Autodesk Inventor part; units mm, degrees
(part 2 of 2)
sketch "スケッチ6" plane through (0, 0, -3) normal (0, 0, -1) x (-1, 0, 0)
  line L0 (6.4129, 87.5325) -> (28.1361, 63.912) projected
  arc A0 (28.2548, 62.7161) -> (28.1361, 63.912) centre (27.4001, 63.2351) ccw projected
  arc A1 (28.2548, 62.7161) -> (28.3025, 54.3338) centre (35.0928, 58.5637) ccw projected
  arc A2 (28.2815, 53.244) -> (28.3025, 54.3338) centre (27.4537, 53.805) ccw projected
  arc A3 (28.2815, 53.244) -> (27.9209, 52.5865) centre (31.5928, 51) ccw projected
  arc A4 (26.9209, 51.9865) -> (27.9209, 52.5865) centre (27.0029, 52.9832) ccw projected
  arc A5 (26.9209, 51.9865) -> (24.1928, 51.2) centre (26.5928, 48) ccw projected
  arc A6 (23.5928, 51) -> (24.1928, 51.2) centre (23.5928, 52) ccw projected
  line L1 (23.5928, 51) -> (-14.9001, 51) projected
  arc A7 (-15.5001, 51.2) -> (-14.9001, 51) centre (-14.9001, 52) ccw projected
  arc A8 (-15.5001, 51.2) -> (-18.2282, 51.9865) centre (-17.9001, 48) ccw projected
  arc A9 (-19.2282, 52.5865) -> (-18.2282, 51.9865) centre (-18.3102, 52.9832) ccw projected
  arc A10 (-19.2282, 52.5865) -> (-20.5352, 54.226) centre (-22.9001, 51) ccw projected
  arc A11 (-20.7229, 55.6596) -> (-20.5352, 54.226) centre (-19.944, 55.0325) ccw projected
  line L2 (-20.7229, 55.6596) -> (4.8979, 87.4826) projected
  arc A12 (6.4129, 87.5325) -> (4.8979, 87.4826) centre (5.6769, 86.8555) ccw projected
  line L3 (3.033, 89.9501) -> (-23.1212, 57.4646) projected
  arc A13 (-24.9001, 58.0917) -> (-23.1212, 57.4646) centre (-23.9001, 58.0917) ccw projected
  line L4 (-24.9001, 58.0917) -> (-24.9001, 116.7814) projected
  arc A14 (-24.1779, 117.742) -> (-24.9001, 116.7814) centre (-23.9001, 116.7814) ccw projected
  arc A15 (-24.1779, 117.742) -> (-22.8335, 118.2662) centre (-26.4001, 125.4272) ccw projected
  arc A16 (-21.6516, 118.048) -> (-22.8335, 118.2662) centre (-22.3876, 117.3711) ccw projected
  line L5 (-21.6516, 118.048) -> (2.9902, 91.2541) projected
  arc A17 (3.033, 89.9501) -> (2.9902, 91.2541) centre (2.2541, 90.5772) ccw projected
  arc A18 (10.5684, 93.4279) -> (14.253, 93.0788) centre (13.05, 100) ccw projected
  arc A19 (15.3071, 92.5632) -> (14.253, 93.0788) centre (14.4242, 92.0935) ccw projected
  line L6 (15.3071, 92.5632) -> (24.5983, 75.0975) projected
  arc A20 (22.9794, 73.9509) -> (24.5983, 75.0975) centre (23.7154, 74.6278) ccw projected
  line L7 (22.9794, 73.9509) -> (8.1117, 90.1171) projected
  arc A21 (8.0688, 91.4211) -> (8.1117, 90.1171) centre (8.8478, 90.794) ccw projected
  line L8 (8.0688, 91.4211) -> (9.4362, 93.1195) projected
  arc A22 (10.5684, 93.4279) -> (9.4362, 93.1195) centre (10.2151, 92.4924) ccw projected
  line L9 (-14.28, 117.3918) -> (-15.0025, 116.7273) projected
  arc A23 (-16.4155, 116.7864) -> (-15.0025, 116.7273) centre (-15.6794, 117.4633) ccw projected
  line L10 (-16.4155, 116.7864) -> (-18.5628, 119.1212) projected
  arc A24 (-17.4982, 120.7426) -> (-18.5628, 119.1212) centre (-17.8267, 119.7981) ccw projected
  line L11 (-17.4982, 120.7426) -> (-14.7786, 119.7967) projected
  arc A25 (-14.1165, 118.9889) -> (-14.7786, 119.7967) centre (-15.1071, 118.8522) ccw projected
  arc A26 (-14.1165, 118.9889) -> (-13.9936, 118.3962) centre (-9.6587, 119.604) ccw projected
  arc A27 (-14.28, 117.3918) -> (-13.9936, 118.3962) centre (-14.9569, 118.1278) ccw projected
  arc A28 (32.5928, 51) -> (30.5928, 51) centre (31.5928, 51) ccw projected
  line L12 (32.5928, 51) -> (37.5928, 51) projected
  arc A29 (39.5928, 51) -> (37.5928, 51) centre (38.5928, 51) ccw projected
  line L13 (39.5928, 51) -> (39.5928, 48) projected
  arc A30 (37.5928, 48) -> (39.5928, 48) centre (38.5928, 48) ccw projected
  line L14 (37.5928, 48) -> (32.5928, 48) projected
  arc A31 (30.5928, 48) -> (32.5928, 48) centre (31.5928, 48) ccw projected
  line L15 (30.5928, 48) -> (30.5928, 51) projected
  circle A32 centre (-9.6587, 119.604) radius 1.5 projected
  circle A33 centre (13.05, 100) radius 4.025 projected
  circle A34 centre (-26.4001, 125.4272) radius 4 projected
  circle A35 centre (35.0928, 58.5637) radius 4 projected
  line L16 (7.0994, 95.0009) -> (6.2039, 93.8886) projected
  arc A36 (4.689, 93.8388) -> (6.2039, 93.8886) centre (5.425, 94.5157) ccw projected
  line L17 (4.689, 93.8388) -> (-13.0309, 113.1062) projected
  arc A37 (-12.9717, 114.5191) -> (-13.0309, 113.1062) centre (-12.2948, 113.7831) ccw projected
  line L18 (-12.9717, 114.5191) -> (-12.2492, 115.1836) projected
  arc A38 (-11.2244, 115.3851) -> (-12.2492, 115.1836) centre (-11.5723, 114.4476) ccw projected
  arc A39 (-11.2244, 115.3851) -> (-7.9613, 115.4364) centre (-9.6587, 119.604) ccw projected
  arc A40 (-6.9306, 115.2672) -> (-7.9613, 115.4364) centre (-7.5841, 114.5103) ccw projected
  line L19 (-6.9306, 115.2672) -> (6.2975, 103.8477) projected
  arc A41 (6.5669, 102.7056) -> (6.2975, 103.8477) centre (5.644, 103.0907) ccw projected
  arc A42 (6.5669, 102.7056) -> (7.1591, 96.1728) centre (13.05, 100) ccw projected
  arc A43 (7.0994, 95.0009) -> (7.1591, 96.1728) centre (6.3205, 95.628) ccw projected
  arc A44 (-28.9001, 51) -> (-30.9001, 51) centre (-29.9001, 51) ccw projected
  line L20 (-28.9001, 51) -> (-23.9001, 51) projected
  arc A45 (-21.9001, 51) -> (-23.9001, 51) centre (-22.9001, 51) ccw projected
  line L21 (-21.9001, 51) -> (-21.9001, 48) projected
  arc A46 (-23.9001, 48) -> (-21.9001, 48) centre (-22.9001, 48) ccw projected
  line L22 (-23.9001, 48) -> (-28.9001, 48) projected
  arc A47 (-30.9001, 48) -> (-28.9001, 48) centre (-29.9001, 48) ccw projected
  line L23 (-30.9001, 48) -> (-30.9001, 51) projected
  line L24 (-27.9001, 116.7814) -> (-27.9001, 55.899) projected
  arc A48 (-29.1001, 54.9192) -> (-27.9001, 55.899) centre (-28.9001, 55.899) ccw projected
  arc A49 (-29.1001, 54.9192) -> (-33.572, 52.5865) centre (-29.9001, 51) ccw projected
  arc A50 (-34.572, 51.9865) -> (-33.572, 52.5865) centre (-34.49, 52.9832) ccw projected
  arc A51 (-34.572, 51.9865) -> (-37.3001, 51.2) centre (-34.9001, 48) ccw projected
  arc A52 (-37.9001, 51) -> (-37.3001, 51.2) centre (-37.9001, 52) ccw projected
  line L25 (-37.9001, 51) -> (-38.9001, 51) projected
  line L26 (-38.9001, 51) -> (-38.9001, 48) projected
  line L27 (-38.9001, 48) -> (-35.9001, 48) projected
  arc A53 (-33.9001, 48) -> (-35.9001, 48) centre (-34.9001, 48) ccw projected
  line L28 (-33.9001, 48) -> (-33.9001, 45) projected
  line L29 (-33.9001, 45) -> (-18.9001, 45) projected
  line L30 (-18.9001, 45) -> (-18.9001, 48) projected
  arc A54 (-16.9001, 48) -> (-18.9001, 48) centre (-17.9001, 48) ccw projected
  line L31 (-16.9001, 48) -> (25.5928, 48) projected
  arc A55 (27.5928, 48) -> (25.5928, 48) centre (26.5928, 48) ccw projected
  line L32 (27.5928, 48) -> (27.5928, 45) projected
  line L33 (27.5928, 45) -> (42.5928, 45) projected
  line L34 (42.5928, 45) -> (42.5928, 48) projected
  arc A56 (44.5928, 48) -> (42.5928, 48) centre (43.5928, 48) ccw projected
  line L35 (44.5928, 48) -> (47.5928, 48) projected
  line L36 (47.5928, 48) -> (47.5928, 51) projected
  line L37 (47.5928, 51) -> (46.5928, 51) projected
  arc A57 (45.9928, 51.2) -> (46.5928, 51) centre (46.5928, 52) ccw projected
  arc A58 (45.9928, 51.2) -> (43.2647, 51.9865) centre (43.5928, 48) ccw projected
  arc A59 (42.2647, 52.5865) -> (43.2647, 51.9865) centre (43.1827, 52.9832) ccw projected
  arc A60 (42.2647, 52.5865) -> (41.904, 53.244) centre (38.5928, 51) ccw projected
  arc A61 (41.883, 54.3338) -> (41.904, 53.244) centre (42.7318, 53.805) ccw projected
  arc A62 (41.883, 54.3338) -> (33.4453, 66.3922) centre (35.0928, 58.5637) ccw projected
  arc A63 (32.3566, 66.9011) -> (33.4453, 66.3922) centre (33.2394, 67.3708) ccw projected
  line L38 (32.3566, 66.9011) -> (17.9557, 93.9721) projected
  arc A64 (18.1172, 95.1344) -> (17.9557, 93.9721) centre (18.8385, 94.4418) ccw projected
  arc A65 (18.1172, 95.1344) -> (9.4271, 106.0187) centre (13.05, 100) ccw projected
  arc A66 (8.2579, 106.1185) -> (9.4271, 106.0187) centre (8.9114, 106.8755) ccw projected
  line L39 (8.2579, 106.1185) -> (-4.9702, 117.5381) projected
  arc A67 (-5.288, 118.533) -> (-4.9702, 117.5381) centre (-4.3167, 118.295) ccw projected
  arc A68 (-5.288, 118.533) -> (-12.7725, 122.8527) centre (-9.6587, 119.604) ccw projected
  arc A69 (-13.793, 122.6301) -> (-12.7725, 122.8527) centre (-13.4645, 123.5746) ccw projected
  line L40 (-13.793, 122.6301) -> (-17.7414, 124.0035) projected
  arc A70 (-18.4115, 125.0013) -> (-17.7414, 124.0035) centre (-17.4129, 124.948) ccw projected
  arc A71 (-18.4115, 125.0013) -> (-28.6223, 117.742) centre (-26.4001, 125.4272) ccw projected
  arc A72 (-27.9001, 116.7814) -> (-28.6223, 117.742) centre (-28.9001, 116.7814) ccw projected
  circle A73 centre (-9.6587, 119.604) radius 1.5 projected
  circle A74 centre (-9.6587, 119.604) radius 3
  point P0 (0, 0)
  dimension "d89" = 6
  constraints: 1 centre point, 1 coincident
  measures "d89" diameter of A74
extrude "押し出し7" cut sketch "スケッチ6" against normal blind 0.6 contours A74
sketch "スケッチ7" plane through (-35.0928, 58.5637, -2.3) normal (0, 0, -1) x (-1, 0, 0)
  arc A0 (6.7903, -4.2299) -> (6.8112, -5.3197) centre (7.6391, -4.7587) ccw projected
  arc A1 (7.1719, -5.9772) -> (6.8112, -5.3197) centre (3.5, -7.5637) ccw projected
  arc A2 (7.1719, -5.9772) -> (8.1719, -6.5772) centre (8.0899, -5.5805) ccw projected
  arc A3 (10.9, -7.3637) -> (8.1719, -6.5772) centre (8.5, -10.5637) ccw projected
  arc A4 (10.9, -7.3637) -> (11.5, -7.5637) centre (11.5, -6.5637) ccw projected
  line L0 (11.5, -7.5637) -> (12.5, -7.5637) projected
  line L1 (12.5, -7.5637) -> (12.5, -10.5637) projected
  line L2 (12.5, -10.5637) -> (9.5, -10.5637) projected
  arc A5 (9.5, -10.5637) -> (7.5, -10.5637) centre (8.5, -10.5637) ccw projected
  line L3 (7.5, -10.5637) -> (7.5, -13.5637) projected
  line L4 (7.5, -13.5637) -> (-7.5, -13.5637) projected
  line L5 (-7.5, -13.5637) -> (-7.5, -10.5637) projected
  arc A6 (-7.5, -10.5637) -> (-9.5, -10.5637) centre (-8.5, -10.5637) ccw projected
  line L6 (-9.5, -10.5637) -> (-51.9929, -10.5637) projected
  arc A7 (-51.9929, -10.5637) -> (-53.9929, -10.5637) centre (-52.9929, -10.5637) ccw projected
  line L7 (-53.9929, -10.5637) -> (-53.9929, -13.5637) projected
  line L8 (-53.9929, -13.5637) -> (-68.9929, -13.5637) projected
  line L9 (-68.9929, -13.5637) -> (-68.9929, -10.5637) projected
  arc A8 (-68.9929, -10.5637) -> (-70.9929, -10.5637) centre (-69.9929, -10.5637) ccw projected
  line L10 (-70.9929, -10.5637) -> (-73.9929, -10.5637) projected
  line L11 (-73.9929, -10.5637) -> (-73.9929, -7.5637) projected
  line L12 (-73.9929, -7.5637) -> (-72.9929, -7.5637) projected
  arc A9 (-72.9929, -7.5637) -> (-72.3929, -7.3637) centre (-72.9929, -6.5637) ccw projected
  arc A10 (-69.6648, -6.5772) -> (-72.3929, -7.3637) centre (-69.9929, -10.5637) ccw projected
  arc A11 (-69.6648, -6.5772) -> (-68.6648, -5.9772) centre (-69.5828, -5.5805) ccw projected
  arc A12 (-64.1929, -3.6445) -> (-68.6648, -5.9772) centre (-64.9929, -7.5637) ccw projected
  arc A13 (-64.1929, -3.6445) -> (-62.9929, -2.6647) centre (-63.9929, -2.6647) ccw projected
  line L13 (-62.9929, -2.6647) -> (-62.9929, 58.2177) projected
  arc A14 (-62.9929, 58.2177) -> (-63.7151, 59.1783) centre (-63.9929, 58.2177) ccw projected
  arc A15 (-53.5042, 66.4376) -> (-63.7151, 59.1783) centre (-61.4929, 66.8635) ccw projected
  arc A16 (-53.5042, 66.4376) -> (-52.8342, 65.4398) centre (-52.5057, 66.3843) ccw projected
  line L14 (-52.8342, 65.4398) -> (-48.8858, 64.0664) projected
  arc A17 (-48.8858, 64.0664) -> (-47.8653, 64.289) centre (-48.5572, 65.0109) ccw projected
  arc A18 (-40.3808, 59.9693) -> (-47.8653, 64.289) centre (-44.7515, 61.0403) ccw projected
  arc A19 (-40.3808, 59.9693) -> (-40.063, 58.9744) centre (-39.4095, 59.7313) ccw projected
  line L15 (-40.063, 58.9744) -> (-26.8349, 47.5548) projected
  arc A20 (-26.8349, 47.5548) -> (-25.6657, 47.455) centre (-26.1814, 48.3118) ccw projected
  arc A21 (-16.9756, 36.5707) -> (-25.6657, 47.455) centre (-22.0428, 41.4363) ccw projected
  arc A22 (-16.9756, 36.5707) -> (-17.1371, 35.4084) centre (-16.2543, 35.8781) ccw projected
  line L16 (-17.1371, 35.4084) -> (-2.7362, 8.3375) projected
  arc A23 (-2.7362, 8.3375) -> (-1.6474, 7.8285) centre (-1.8534, 8.8071) ccw projected
  arc A24 (6.7903, -4.2299) -> (-1.6474, 7.8285) centre (0, 0) ccw projected
  arc A25 (-24.5244, 34.8642) -> (-25.6566, 34.5558) centre (-24.8776, 33.9287) ccw projected
  line L17 (-25.6566, 34.5558) -> (-27.0239, 32.8574) projected
  arc A26 (-27.0239, 32.8574) -> (-26.9811, 31.5534) centre (-26.245, 32.2303) ccw projected
  line L18 (-26.9811, 31.5534) -> (-12.1134, 15.3872) projected
  arc A27 (-12.1134, 15.3872) -> (-10.4945, 16.5338) centre (-11.3773, 16.0642) ccw projected
  line L19 (-10.4945, 16.5338) -> (-19.7857, 33.9995) projected
  arc A28 (-19.7857, 33.9995) -> (-20.8398, 34.5151) centre (-20.6685, 33.5298) ccw projected
  arc A29 (-24.5244, 34.8642) -> (-20.8398, 34.5151) centre (-22.0428, 41.4363) ccw projected
  arc A30 (-59.2707, 59.1783) -> (-59.9929, 58.2177) centre (-58.9929, 58.2177) ccw projected
  line L20 (-59.9929, 58.2177) -> (-59.9929, -0.472) projected
  arc A31 (-59.9929, -0.472) -> (-58.214, -1.0991) centre (-58.9929, -0.472) ccw projected
  line L21 (-58.214, -1.0991) -> (-32.0597, 31.3864) projected
  arc A32 (-32.0597, 31.3864) -> (-32.1026, 32.6904) centre (-32.8387, 32.0135) ccw projected
  line L22 (-32.1026, 32.6904) -> (-56.7444, 59.4843) projected
  arc A33 (-56.7444, 59.4843) -> (-57.9263, 59.7025) centre (-57.4804, 58.8074) ccw projected
  arc A34 (-59.2707, 59.1783) -> (-57.9263, 59.7025) centre (-61.4929, 66.8635) ccw projected
  arc A35 (-28.6799, 28.9688) -> (-30.1948, 28.9189) centre (-29.4159, 28.2918) ccw projected
  line L23 (-30.1948, 28.9189) -> (-55.8157, -2.9041) projected
  arc A36 (-55.8157, -2.9041) -> (-55.628, -4.3377) centre (-55.0367, -3.5312) ccw projected
  arc A37 (-54.321, -5.9772) -> (-55.628, -4.3377) centre (-57.9929, -7.5637) ccw projected
  arc A38 (-54.321, -5.9772) -> (-53.321, -6.5772) centre (-53.403, -5.5805) ccw projected
  arc A39 (-50.5929, -7.3637) -> (-53.321, -6.5772) centre (-52.9929, -10.5637) ccw projected
  arc A40 (-50.5929, -7.3637) -> (-49.9929, -7.5637) centre (-49.9929, -6.5637) ccw projected
  line L24 (-49.9929, -7.5637) -> (-11.5, -7.5637) projected
  arc A41 (-11.5, -7.5637) -> (-10.9, -7.3637) centre (-11.5, -6.5637) ccw projected
  arc A42 (-8.1719, -6.5772) -> (-10.9, -7.3637) centre (-8.5, -10.5637) ccw projected
  arc A43 (-8.1719, -6.5772) -> (-7.1719, -5.9772) centre (-8.0899, -5.5805) ccw projected
  arc A44 (-6.8112, -5.3197) -> (-7.1719, -5.9772) centre (-3.5, -7.5637) ccw projected
  arc A45 (-6.8112, -5.3197) -> (-6.7903, -4.2299) centre (-7.6391, -4.7587) ccw projected
  arc A46 (-6.838, 4.1524) -> (-6.7903, -4.2299) centre (0, 0) ccw projected
  arc A47 (-6.838, 4.1524) -> (-6.9567, 5.3483) centre (-7.6927, 4.6714) ccw projected
  line L25 (-6.9567, 5.3483) -> (-28.6799, 28.9688) projected
  line L26 (2.5, -7.5637) -> (-2.5, -7.5637) projected
  arc A48 (-2.5, -7.5637) -> (-4.5, -7.5637) centre (-3.5, -7.5637) ccw projected
  line L27 (-4.5, -7.5637) -> (-4.5, -10.5637) projected
  arc A49 (-4.5, -10.5637) -> (-2.5, -10.5637) centre (-3.5, -10.5637) ccw projected
  line L28 (-2.5, -10.5637) -> (2.5, -10.5637) projected
  arc A50 (2.5, -10.5637) -> (4.5, -10.5637) centre (3.5, -10.5637) ccw projected
  line L29 (4.5, -10.5637) -> (4.5, -7.5637) projected
  arc A51 (4.5, -7.5637) -> (2.5, -7.5637) centre (3.5, -7.5637) ccw projected
  line L30 (-58.9929, -7.5637) -> (-63.9929, -7.5637) projected
  arc A52 (-63.9929, -7.5637) -> (-65.9929, -7.5637) centre (-64.9929, -7.5637) ccw projected
  line L31 (-65.9929, -7.5637) -> (-65.9929, -10.5637) projected
  arc A53 (-65.9929, -10.5637) -> (-63.9929, -10.5637) centre (-64.9929, -10.5637) ccw projected
  line L32 (-63.9929, -10.5637) -> (-58.9929, -10.5637) projected
  arc A54 (-58.9929, -10.5637) -> (-56.9929, -10.5637) centre (-57.9929, -10.5637) ccw projected
  line L33 (-56.9929, -10.5637) -> (-56.9929, -7.5637) projected
  arc A55 (-56.9929, -7.5637) -> (-58.9929, -7.5637) centre (-57.9929, -7.5637) ccw projected
  arc A56 (-46.3171, 56.8214) -> (-47.342, 56.6199) centre (-46.665, 55.8839) ccw projected
  line L34 (-47.342, 56.6199) -> (-48.0645, 55.9554) projected
  arc A57 (-48.0645, 55.9554) -> (-48.1236, 54.5425) centre (-47.3876, 55.2194) ccw projected
  line L35 (-48.1236, 54.5425) -> (-30.4038, 35.2751) projected
  arc A58 (-30.4038, 35.2751) -> (-28.8888, 35.3249) centre (-29.6678, 35.952) ccw projected
  line L36 (-28.8888, 35.3249) -> (-27.9933, 36.4372) projected
  arc A59 (-27.9933, 36.4372) -> (-27.9337, 37.6091) centre (-28.7723, 37.0643) ccw projected
  arc A60 (-28.5259, 44.1419) -> (-27.9337, 37.6091) centre (-22.0428, 41.4363) ccw projected
  arc A61 (-28.5259, 44.1419) -> (-28.7953, 45.284) centre (-29.4487, 44.527) ccw projected
  line L37 (-28.7953, 45.284) -> (-42.0234, 56.7035) projected
  arc A62 (-42.0234, 56.7035) -> (-43.054, 56.8727) centre (-42.6768, 55.9466) ccw projected
  arc A63 (-46.3171, 56.8214) -> (-43.054, 56.8727) centre (-44.7515, 61.0403) ccw projected
  arc A64 (-52.591, 62.1789) -> (-53.6555, 60.5575) centre (-52.9195, 61.2344) ccw projected
  line L38 (-53.6555, 60.5575) -> (-51.5083, 58.2227) projected
  arc A65 (-51.5083, 58.2227) -> (-50.0953, 58.1636) centre (-50.7722, 58.8996) ccw projected
  line L39 (-50.0953, 58.1636) -> (-49.3728, 58.8281) projected
  arc A66 (-49.3728, 58.8281) -> (-49.0864, 59.8325) centre (-50.0497, 59.5641) ccw projected
  arc A67 (-49.2092, 60.4252) -> (-49.0864, 59.8325) centre (-44.7515, 61.0403) ccw projected
  arc A68 (-49.2092, 60.4252) -> (-49.8713, 61.233) centre (-50.1999, 60.2885) ccw projected
  line L40 (-49.8713, 61.233) -> (-52.591, 62.1789) projected
  circle A69 centre (0, 0) radius 4 projected
  circle A70 centre (-61.4929, 66.8635) radius 4 projected
  circle A71 centre (-61.4929, 66.8635) radius 2 projected
  circle A72 centre (0, 0) radius 2 projected
  circle A73 centre (-22.0428, 41.4363) radius 4.025 projected
  circle A74 centre (-44.7515, 61.0403) radius 1.5 projected
  point P0 (-35.0928, -58.5637)
extrude "押し出し8" cut sketch "スケッチ7" against normal blind 0.5 contours A69 | A70
sketch "スケッチ8" plane through (0, 0, -3) normal (0, 0, -1) x (-1, 0, 0)
  circle A0 centre (-9.6587, 119.604) radius 3 projected
  arc A1 (41.883, 54.3338) -> (41.904, 53.244) centre (42.7318, 53.805) ccw projected
  arc A2 (42.2647, 52.5865) -> (41.904, 53.244) centre (38.5928, 51) ccw projected
  arc A3 (42.2647, 52.5865) -> (43.2647, 51.9865) centre (43.1827, 52.9832) ccw projected
  arc A4 (45.9928, 51.2) -> (43.2647, 51.9865) centre (43.5928, 48) ccw projected
  arc A5 (45.9928, 51.2) -> (46.5928, 51) centre (46.5928, 52) ccw projected
  line L0 (46.5928, 51) -> (47.5928, 51) projected
  line L1 (47.5928, 51) -> (47.5928, 48) projected
  line L2 (47.5928, 48) -> (44.5928, 48) projected
  arc A6 (44.5928, 48) -> (42.5928, 48) centre (43.5928, 48) ccw projected
  line L3 (42.5928, 48) -> (42.5928, 45) projected
  line L4 (42.5928, 45) -> (27.5928, 45) projected
  line L5 (27.5928, 45) -> (27.5928, 48) projected
  arc A7 (27.5928, 48) -> (25.5928, 48) centre (26.5928, 48) ccw projected
  line L6 (25.5928, 48) -> (-16.9001, 48) projected
  arc A8 (-16.9001, 48) -> (-18.9001, 48) centre (-17.9001, 48) ccw projected
  line L7 (-18.9001, 48) -> (-18.9001, 45) projected
  line L8 (-18.9001, 45) -> (-33.9001, 45) projected
  line L9 (-33.9001, 45) -> (-33.9001, 48) projected
  arc A9 (-33.9001, 48) -> (-35.9001, 48) centre (-34.9001, 48) ccw projected
  line L10 (-35.9001, 48) -> (-38.9001, 48) projected
  line L11 (-38.9001, 48) -> (-38.9001, 51) projected
  line L12 (-38.9001, 51) -> (-37.9001, 51) projected
  arc A10 (-37.9001, 51) -> (-37.3001, 51.2) centre (-37.9001, 52) ccw projected
  arc A11 (-34.572, 51.9865) -> (-37.3001, 51.2) centre (-34.9001, 48) ccw projected
  arc A12 (-34.572, 51.9865) -> (-33.572, 52.5865) centre (-34.49, 52.9832) ccw projected
  arc A13 (-29.1001, 54.9192) -> (-33.572, 52.5865) centre (-29.9001, 51) ccw projected
  arc A14 (-29.1001, 54.9192) -> (-27.9001, 55.899) centre (-28.9001, 55.899) ccw projected
  line L13 (-27.9001, 55.899) -> (-27.9001, 116.7814) projected
  arc A15 (-27.9001, 116.7814) -> (-28.6223, 117.742) centre (-28.9001, 116.7814) ccw projected
  arc A16 (-18.4115, 125.0013) -> (-28.6223, 117.742) centre (-26.4001, 125.4272) ccw projected
  arc A17 (-18.4115, 125.0013) -> (-17.7414, 124.0035) centre (-17.4129, 124.948) ccw projected
  line L14 (-17.7414, 124.0035) -> (-13.793, 122.6301) projected
  arc A18 (-13.793, 122.6301) -> (-12.7725, 122.8527) centre (-13.4645, 123.5746) ccw projected
  arc A19 (-5.288, 118.533) -> (-12.7725, 122.8527) centre (-9.6587, 119.604) ccw projected
  arc A20 (-5.288, 118.533) -> (-4.9702, 117.5381) centre (-4.3167, 118.295) ccw projected
  line L15 (-4.9702, 117.5381) -> (8.2579, 106.1185) projected
  arc A21 (8.2579, 106.1185) -> (9.4271, 106.0187) centre (8.9114, 106.8755) ccw projected
  arc A22 (18.1172, 95.1344) -> (9.4271, 106.0187) centre (13.05, 100) ccw projected
  arc A23 (18.1172, 95.1344) -> (17.9557, 93.9721) centre (18.8385, 94.4418) ccw projected
  line L16 (17.9557, 93.9721) -> (32.3566, 66.9011) projected
  arc A24 (32.3566, 66.9011) -> (33.4453, 66.3922) centre (33.2394, 67.3708) ccw projected
  arc A25 (41.883, 54.3338) -> (33.4453, 66.3922) centre (35.0928, 58.5637) ccw projected
  arc A26 (10.5684, 93.4279) -> (9.4362, 93.1195) centre (10.2151, 92.4924) ccw projected
  line L17 (9.4362, 93.1195) -> (8.0688, 91.4211) projected
  arc A27 (8.0688, 91.4211) -> (8.1117, 90.1171) centre (8.8478, 90.794) ccw projected
  line L18 (8.1117, 90.1171) -> (22.9794, 73.9509) projected
  arc A28 (22.9794, 73.9509) -> (24.5983, 75.0975) centre (23.7154, 74.6278) ccw projected
  line L19 (24.5983, 75.0975) -> (15.3071, 92.5632) projected
  arc A29 (15.3071, 92.5632) -> (14.253, 93.0788) centre (14.4242, 92.0935) ccw projected
  arc A30 (10.5684, 93.4279) -> (14.253, 93.0788) centre (13.05, 100) ccw projected
  arc A31 (-24.1779, 117.742) -> (-24.9001, 116.7814) centre (-23.9001, 116.7814) ccw projected
  line L20 (-24.9001, 116.7814) -> (-24.9001, 58.0917) projected
  arc A32 (-24.9001, 58.0917) -> (-23.1212, 57.4646) centre (-23.9001, 58.0917) ccw projected
  line L21 (-23.1212, 57.4646) -> (3.033, 89.9501) projected
  arc A33 (3.033, 89.9501) -> (2.9902, 91.2541) centre (2.2541, 90.5772) ccw projected
  line L22 (2.9902, 91.2541) -> (-21.6516, 118.048) projected
  arc A34 (-21.6516, 118.048) -> (-22.8335, 118.2662) centre (-22.3876, 117.3711) ccw projected
  arc A35 (-24.1779, 117.742) -> (-22.8335, 118.2662) centre (-26.4001, 125.4272) ccw projected
  arc A36 (6.4129, 87.5325) -> (4.8979, 87.4826) centre (5.6769, 86.8555) ccw projected
  line L23 (4.8979, 87.4826) -> (-20.7229, 55.6596) projected
  arc A37 (-20.7229, 55.6596) -> (-20.5352, 54.226) centre (-19.944, 55.0325) ccw projected
  arc A38 (-19.2282, 52.5865) -> (-20.5352, 54.226) centre (-22.9001, 51) ccw projected
  arc A39 (-19.2282, 52.5865) -> (-18.2282, 51.9865) centre (-18.3102, 52.9832) ccw projected
  arc A40 (-15.5001, 51.2) -> (-18.2282, 51.9865) centre (-17.9001, 48) ccw projected
  arc A41 (-15.5001, 51.2) -> (-14.9001, 51) centre (-14.9001, 52) ccw projected
  line L24 (-14.9001, 51) -> (23.5928, 51) projected
  arc A42 (23.5928, 51) -> (24.1928, 51.2) centre (23.5928, 52) ccw projected
  arc A43 (26.9209, 51.9865) -> (24.1928, 51.2) centre (26.5928, 48) ccw projected
  arc A44 (26.9209, 51.9865) -> (27.9209, 52.5865) centre (27.0029, 52.9832) ccw projected
  arc A45 (28.2815, 53.244) -> (27.9209, 52.5865) centre (31.5928, 51) ccw projected
  arc A46 (28.2815, 53.244) -> (28.3025, 54.3338) centre (27.4537, 53.805) ccw projected
  arc A47 (28.2548, 62.7161) -> (28.3025, 54.3338) centre (35.0928, 58.5637) ccw projected
  arc A48 (28.2548, 62.7161) -> (28.1361, 63.912) centre (27.4001, 63.2351) ccw projected
  line L25 (28.1361, 63.912) -> (6.4129, 87.5325) projected
  line L26 (37.5928, 51) -> (32.5928, 51) projected
  arc A49 (32.5928, 51) -> (30.5928, 51) centre (31.5928, 51) ccw projected
  line L27 (30.5928, 51) -> (30.5928, 48) projected
  arc A50 (30.5928, 48) -> (32.5928, 48) centre (31.5928, 48) ccw projected
  line L28 (32.5928, 48) -> (37.5928, 48) projected
  arc A51 (37.5928, 48) -> (39.5928, 48) centre (38.5928, 48) ccw projected
  line L29 (39.5928, 48) -> (39.5928, 51) projected
  arc A52 (39.5928, 51) -> (37.5928, 51) centre (38.5928, 51) ccw projected
  line L30 (-23.9001, 51) -> (-28.9001, 51) projected
  arc A53 (-28.9001, 51) -> (-30.9001, 51) centre (-29.9001, 51) ccw projected
  line L31 (-30.9001, 51) -> (-30.9001, 48) projected
  arc A54 (-30.9001, 48) -> (-28.9001, 48) centre (-29.9001, 48) ccw projected
  line L32 (-28.9001, 48) -> (-23.9001, 48) projected
  arc A55 (-23.9001, 48) -> (-21.9001, 48) centre (-22.9001, 48) ccw projected
  line L33 (-21.9001, 48) -> (-21.9001, 51) projected
  arc A56 (-21.9001, 51) -> (-23.9001, 51) centre (-22.9001, 51) ccw projected
  arc A57 (-11.2244, 115.3851) -> (-12.2492, 115.1836) centre (-11.5723, 114.4476) ccw projected
  line L34 (-12.2492, 115.1836) -> (-12.9717, 114.5191) projected
  arc A58 (-12.9717, 114.5191) -> (-13.0309, 113.1062) centre (-12.2948, 113.7831) ccw projected
  line L35 (-13.0309, 113.1062) -> (4.689, 93.8388) projected
  arc A59 (4.689, 93.8388) -> (6.2039, 93.8886) centre (5.425, 94.5157) ccw projected
  line L36 (6.2039, 93.8886) -> (7.0994, 95.0009) projected
  arc A60 (7.0994, 95.0009) -> (7.1591, 96.1728) centre (6.3205, 95.628) ccw projected
  arc A61 (6.5669, 102.7056) -> (7.1591, 96.1728) centre (13.05, 100) ccw projected
  arc A62 (6.5669, 102.7056) -> (6.2975, 103.8477) centre (5.644, 103.0907) ccw projected
  line L37 (6.2975, 103.8477) -> (-6.9306, 115.2672) projected
  arc A63 (-6.9306, 115.2672) -> (-7.9613, 115.4364) centre (-7.5841, 114.5103) ccw projected
  arc A64 (-11.2244, 115.3851) -> (-7.9613, 115.4364) centre (-9.6587, 119.604) ccw projected
  arc A65 (-17.4982, 120.7426) -> (-18.5628, 119.1212) centre (-17.8267, 119.7981) ccw projected
  line L38 (-18.5628, 119.1212) -> (-16.4155, 116.7864) projected
  arc A66 (-16.4155, 116.7864) -> (-15.0025, 116.7273) centre (-15.6794, 117.4633) ccw projected
  line L39 (-15.0025, 116.7273) -> (-14.28, 117.3918) projected
  arc A67 (-14.28, 117.3918) -> (-13.9936, 118.3962) centre (-14.9569, 118.1278) ccw projected
  arc A68 (-14.1165, 118.9889) -> (-13.9936, 118.3962) centre (-9.6587, 119.604) ccw projected
  arc A69 (-14.1165, 118.9889) -> (-14.7786, 119.7967) centre (-15.1071, 118.8522) ccw projected
  line L40 (-14.7786, 119.7967) -> (-17.4982, 120.7426) projected
  circle A70 centre (35.0928, 58.5637) radius 4 projected
  circle A71 centre (-26.4001, 125.4272) radius 4 projected
  circle A72 centre (13.05, 100) radius 4.025 projected
  circle A73 centre (-9.6587, 119.604) radius 1.5 projected
  point P0 (0, 0)
extrude "押し出し9" add sketch "スケッチ8" against normal blind 3 contours A0
